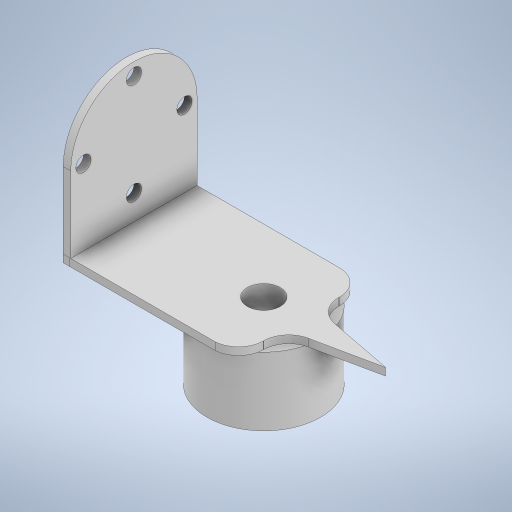
# Autodesk Inventor part: Herramienta
Saved by Autodesk Inventor 2023 (Build 270158000, 158)
## iProperties
Created: 2023-05-31
Part Number: Herramienta
Material: Genérico
Document SubType Name: Modeling
Designer: Jhon Cáceres
Density: 1 g/cm^3
Appearance: Valor por defecto
Author: Jhon Cáceres
Autodesk Inventor part; units mm, degrees
ref_plane "YZ Plane" through (0, 0, 0) normal (1, 0, 0) x (0, 1, 0)
ref_plane "XZ Plane" through (0, 0, 0) normal (0, 1, 0) x (-1, 0, 0)
ref_plane "XY Plane" through (0, 0, 0) normal (0, 0, 1) x (1, 0, 0)
sketch "Boceto1" plane through (0, 0, 0) normal (1, 0, 0) x (0, 1, 0)
  circle A0 centre (0, 0) radius 25
  circle A1 centre (0, 0) radius 20
  circle A2 centre (20, 0) radius 3
  circle A3 centre (0, 20) radius 3
  circle A4 centre (-20, 0) radius 3
  circle A5 centre (0, -20) radius 3
  line L0 (0, 25) -> (-31.5, 25)
  line L1 (-31.5, 25) -> (-31.5, -25)
  line L2 (-31.5, -25) -> (0, -25)
  line L3 (0, -25) -> (0, 25)
  point P0 (0, -25)
  dimension "d1" = 40
  dimension "d0" = 50
  dimension "d2" = 6
  dimension "d5" = 360
  dimension "d7" = 31.5
  dimension "d8" = 0
  dimension "d9" = 50
  dimension "d10" = 25
  constraints: 8 end point, 5 centre point, 2 coincident, 2 parallel, 1 horizontal, 1 horizontal alignment, 1 perpendicular, 11 other
  measures "d0" diameter of A0
  measures "d2" diameter of A2
  measures "d7" distance of L0.start L0.end
  measures "d8" distance from line of A3.centre L3
  measures "d9" distance of L2.end L0.start
  measures "d10" distance from line of point (0, 0) L2
extrude "Extrusión1" add sketch "Boceto1" along normal blind 3 contours A0 L3 A5 A1 A2 A3 | L3 A3 A1 A4 A5 A0 | A0 L2 L1 L0 | A3 L3 A5 A1 A4 | A1 A2 A5 L3 A3
sketch "Boceto2" plane through (3, 0, 0) normal (1, 0, 0) x (0, 0, -1)
  line L0 (25, -30) -> (-25, -30)
  line L1 (-25, -30) -> (-25, -33)
  line L2 (-25, -33) -> (25, -33)
  line L3 (25, -33) -> (25, -30)
  line L4 (-25, -31.5) -> (25, -31.5) projected
  point P0 (0, 0)
  dimension "d13" = 50
  dimension "d14" = 3
  dimension "d15" = 1.5
  constraints: 8 end point, 2 parallel, 1 horizontal, 1 perpendicular
  measures "d13" distance of L2.end L1.end
  measures "d14" distance of L2.end L0.start
  measures "d15" distance between parallel lines of L4 L2
extrude "Extrusión2" add sketch "Boceto2" along normal blind 100
sketch "Boceto3" plane through (3, 0, 0) normal (-1, 0, 0) x (0, 0, 1)
  line L0 (25, -31.5) -> (-25, -31.5) projected
  line L1 (-25, -33) -> (-25, -31.5) projected
  line L2 (25, -31.5) -> (-25, -31.5)
  line L3 (-25, -31.5) -> (-25, -33)
  line L4 (-25, -33) -> (25, -33)
  line L5 (25, -33) -> (25, -31.5)
  point P0 (0, 0)
  constraints: 8 end point, 2 parallel, 1 horizontal, 1 perpendicular
extrude "Extrusión3" add sketch "Boceto3" along normal blind 3
sketch "Boceto4" plane through (3, -30, 25) normal (0, 1, 0) x (1, 0, 0)
  line L0 (-3.5591, -0.0033) -> (56.4409, -0.0243)
  line L1 (56.4583, 49.9757) -> (-83.1198, 50.0244)
  circle A0 centre (51.4496, 24.9772) radius 6.5
  arc A1 (56.4409, -0.0243) -> (66.4443, 9.9722) centre (56.4443, 9.9757) ccw
  arc A2 (66.4548, 39.9722) -> (56.4583, 49.9757) centre (56.4548, 39.9757) ccw
  line L2 (-3.5591, -0.0033) -> (-0.5591, -0.0044)
  line L3 (-0.5591, -0.0044) -> (-0.5417, 49.9956)
  line L4 (-0.5417, 49.9956) -> (-3.5417, 49.9967)
  line L5 (-3.5581, 2.9967) -> (-0.5581, 2.9956)
  line L6 (-3.557, 5.9967) -> (-0.557, 5.9956)
  line L7 (-3.556, 8.9967) -> (-0.556, 8.9956)
  line L8 (-3.555, 11.9967) -> (-0.555, 11.9956)
  line L9 (-3.5539, 14.9967) -> (-0.5539, 14.9956)
  line L10 (-3.5529, 17.9967) -> (-0.5529, 17.9956)
  line L11 (-3.5518, 20.9967) -> (-0.5518, 20.9956)
  line L12 (-3.5508, 23.9967) -> (-0.5508, 23.9956)
  line L13 (-3.5497, 26.9967) -> (-0.5497, 26.9956)
  line L14 (-3.5487, 29.9967) -> (-0.5487, 29.9956)
  line L15 (-3.5476, 32.9967) -> (-0.5476, 32.9956)
  line L16 (-3.5466, 35.9967) -> (-0.5466, 35.9956)
  line L17 (-3.5455, 38.9967) -> (-0.5455, 38.9956)
  line L18 (-3.5445, 41.9967) -> (-0.5445, 41.9956)
  line L19 (-3.5434, 44.9967) -> (-0.5434, 44.9956)
  line L20 (-3.5424, 47.9967) -> (-0.5424, 47.9956)
  line L21 (-3.5413, 50.9967) -> (-0.5413, 50.9956)
  line L22 (-3.5403, 53.9967) -> (-0.5403, 53.9956)
  line L23 (-3.5392, 56.9967) -> (-0.5392, 56.9956)
  line L24 (-3.5382, 59.9967) -> (-0.5382, 59.9956)
  line L25 (74.533, 29.8898) -> (99.7047, 24.9606)
  line L26 (99.7047, 24.9606) -> (74.3879, 19.6408)
  line L27 (66.4443, 9.9722) -> (66.4443, 9.858)
  line L28 (66.4547, 39.7069) -> (66.4548, 39.9722)
  arc A3 (74.3879, 19.6408) -> (66.4443, 9.858) centre (76.4443, 9.8545) ccw
  arc A4 (66.4547, 39.7069) -> (74.533, 29.8898) centre (76.4547, 39.7034) ccw
  line L29 (0, 50) -> (100, 50) projected
  line L30 (0, 0) -> (100, 0) projected
  circle A5 centre (51.4496, 24.9772) radius 79.9654
  point P0 (-3, 25)
  point P1 (-13.1198, 50)
  point P2 (66.4518, 31.4722)
  point P3 (66.4471, 17.9722)
  dimension "d24" = 70
  dimension "d25" = 13
  dimension "d26" = 10
  dimension "d27" = 3
  dimension "d28" = 3
  dimension "d29" = 7.005
  dimension "d30" = 6.495
  dimension "d31" = 10
  dimension "d33" = 0
  dimension "d34" = 179.98
  constraints: 58 end point, 10 tangent, 8 point on circle, 7 point on line, 6 centre point, 4 perpendicular, 2 equal radius, 2 parallel, 1 coincident, 58 other
  measures "d24" distance of point (-13.12, 50) L1.end
  measures "d25" diameter of A0
  measures "d26" radius of A1
  measures "d27" distance between parallel lines of L5 L2
  measures "d28" distance of L5.start L6.start
  measures "d29" vertical distance of point (66.447, 17.972) A0.centre
  measures "d30" vertical distance of A0.centre point (66.452, 31.472)
  measures "d31" radius of A3
  measures "d33" distance from line of L29 point (-13.12, 50)
  measures "d34" angle of L30 L0
extrude "Extrusión4" cut sketch "Boceto4" against normal blind 3
sketch "Boceto6" plane through (59.4583, -33, -24.9757) normal (0.0003491, 0, -0.9999999) x (-0.9999999, 0, -0.0003491)
  line L0 (57, 0) -> (-0.7, 0) projected
  line L1 (56.4583, 3) -> (59.4583, 3) projected
  line L2 (57, 0) -> (59.4583, 0)
  line L3 (59.4583, 0) -> (59.4583, 3)
  line L4 (59.4583, 3) -> (57, 3)
  line L5 (57, 3) -> (57, 0)
  point P0 (59.4496, 33)
  constraints: 8 end point, 2 parallel, 1 horizontal, 1 perpendicular
extrude "Extrusión5" add sketch "Boceto6" against normal blind 50
sketch "Boceto7" plane through (2.4409, -33, 25) normal (0, -1, 0) x (1, 0, 0)
  circle A0 centre (52.0087, -24.9772) radius 6.5 projected
  circle A1 centre (52.0087, -24.9772) radius 22.5
  point P0 (-2.4409, -25)
  dimension "d39" = 45
  constraints: 1 centre point, 1 coincident
  measures "d39" diameter of A1
extrude "Extrusión6" add sketch "Boceto7" along normal blind 27
